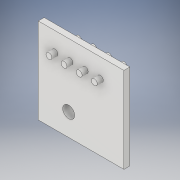
# Autodesk Inventor part: Mic_breakout
Saved by Autodesk Inventor 2018 (Build 220112000, 112)
## iProperties
Created: 2018-06-16
Part Number: Mic_breakout
Material: ABS-Kunststoff
Document SubType Name: Modeling
Designer: ich
Density: 1.06 g/cm^3
Appearance: Glatt - weiß
Author: ich
Autodesk Inventor part; units mm, degrees
note: some values were not read from the file. Chosen so that the rebuilt part matches the saved one: direction of "Bohrung1".
ref_plane "YZ Plane" through (0, 0, 0) normal (1, 0, 0) x (0, 1, 0)
ref_plane "XZ Plane" through (0, 0, 0) normal (0, 1, 0) x (-1, 0, 0)
ref_plane "XY Plane" through (0, 0, 0) normal (0, 0, 1) x (1, 0, 0)
sketch "Skizze1" plane through (0, 0, 0) normal (0, 1, 0) x (-1, 0, 0)
  line L0 (0, 0) -> (14.4, 0)
  line L1 (14.4, 0) -> (14.4, -14.4)
  line L2 (14.4, -14.4) -> (0, -14.4)
  line L3 (0, -14.4) -> (0, 0)
  dimension "d0" = 14.4
  dimension "d1" = 14.4
  constraints: 8 end point, 2 parallel, 1 horizontal, 1 perpendicular
  measures "d0" distance of L1.end L2.end
  measures "d1" distance of L0.end L1.end
extrude "Extrusion1" add sketch "Skizze1" along normal blind 1
sketch "Skizze2" plane through (0, 1, 0) normal (0, 1, 0) x (1, 0, 0)
  line L0 (0, 14.4) -> (-14.4, 14.4) projected
  line L1 (0, 0) -> (0, 14.4) projected
  point P0 (-9.28, 10.68)
  dimension "d4" = 3.72
  dimension "d5" = 9.28
  measures "d4" distance from line of L0 point (-9.28, 10.68)
  measures "d5" distance from line of L1 point (-9.28, 10.68)
hole "Bohrung1" at (-9.28, 1, -10.68) direction (0, -1, 0) diameter 2 end up to surface
sketch "Skizze3" plane through (0, 1, 0) normal (0, 1, 0) x (1, 0, 0)
  circle A0 centre (-9.28, 10.68) radius 1 projected
  line L0 (-14.4, 0) -> (0, 0) projected
  line L1 (0, 0) -> (0, 14.4) projected
  line L2 (0, 14.4) -> (-14.4, 14.4) projected
  line L3 (-14.4, 14.4) -> (-14.4, 0) projected
  line L4 (-10.78, 8) -> (-7.78, 8)
  line L5 (-7.78, 8) -> (-7.78, 12)
  line L6 (-7.78, 12) -> (-10.78, 12)
  line L7 (-10.78, 12) -> (-10.78, 8)
  dimension "d13" = 4
  dimension "d14" = 3
  dimension "d15" = 1.5
  dimension "d16" = 1.32
  constraints: 8 end point, 2 parallel, 1 horizontal, 1 perpendicular
  measures "d13" distance of L6.end L4.start
  measures "d14" distance of L5.end L6.end
  measures "d15" distance from line of L7 A0.centre
  measures "d16" distance from line of L6 A0.centre
extrude "Extrusion2" add sketch "Skizze3" along normal blind 1.2 contours L7 L6 L5 L4
sketch "Skizze4" plane through (0, 1, 0) normal (0, 1, 0) x (1, 0, 0)
  line L0 (-14.4, 14.4) -> (-14.4, 0) construction
  line L1 (-14.4, 3.2) -> (0, 3.2) construction
  line L2 (0, 0) -> (0, 14.4) construction
  line L3 (-14.4, 0) -> (0, 0) projected
  circle A0 centre (-11.6, 3.2) radius 0.5
  circle A1 centre (-9.06, 3.2) radius 0.5
  circle A2 centre (-6.52, 3.2) radius 0.5
  circle A3 centre (-3.98, 3.2) radius 0.5
  dimension "d19" = 3.2
  dimension "d20" = 2.8
  dimension "d21" = 2.54
  dimension "d22" = 2.54
  dimension "d23" = 2.54
  dimension "d24" = 1
  dimension "d25" = 1
  dimension "d26" = 1
  dimension "d27" = 1
  constraints: 6 point on line, 4 centre point, 4 coincident, 2 end point, 1 horizontal
  measures "d19" distance between parallel lines of L3 L1
  measures "d20" distance from line of L0 point (-11.6, 3.2)
  measures "d21" distance of point (-11.6, 3.2) point (-9.06, 3.2)
  measures "d22" distance of point (-6.52, 3.2) point (-9.06, 3.2)
  measures "d23" distance of point (-6.52, 3.2) point (-3.98, 3.2)
  measures "d24" diameter of A0
  measures "d25" diameter of A1
  measures "d26" diameter of A2
  measures "d27" diameter of A3
extrude "Extrusion3" add sketch "Skizze4" along normal blind 3 and the other way blind 2
